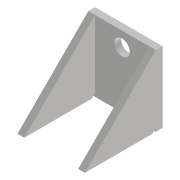
# Autodesk Inventor part: Break_tensor_support
Saved by Autodesk Inventor 2020 (Build 240168000, 168)
## iProperties
Created: 2020-02-19
Part Number: Break_tensor_support
Material: Generic
Document SubType Name: Sheet Metal
Designer: Charlie
Density: 1 g/cm^3
Sheet Metal Rule: Default_mm
Appearance: Default
Mass: 45.5555 g
Surface Area: 194.795 cm^2
Volume: 45.5555 cm^3
Author: Charlie
Autodesk Inventor part; units mm, degrees
ref_plane "YZ Plane" through (0, 0, 0) normal (1, 0, 0) x (0, 1, 0)
ref_plane "XZ Plane" through (0, 0, 0) normal (0, 1, 0) x (-1, 0, 0)
ref_plane "XY Plane" through (0, 0, 0) normal (0, 0, 1) x (1, 0, 0)
sketch "Sketch1" plane through (0, 0, 0) normal (0, 0, 1) x (1, 0, 0)
  circle A0 centre (0, 0) radius 6.85
  line L0 (-30, 13) -> (30, 13)
  line L1 (30, 13) -> (30, -50)
  line L2 (30, -50) -> (-30, -50)
  line L3 (-30, -50) -> (-30, 13)
  point P0 (0, 13)
  dimension "d0" = 13.7
  dimension "d1" = 50
  dimension "d2" = 60
  dimension "d4" = 13
  measures "d0" diameter of A0
  measures "d1" distance from line of L2 point (0, 0)
  measures "d2" distance of L0.start L0.end
  measures "d4" distance from line of L0 point (0, 0)
extrude "Plate1" add sketch "Sketch1" along normal blind 6
sketch "Sketch2" plane through (30, -50, 0) normal (1, 0, 0) x (0, 0, -1)
  line L0 (-6, 63) -> (-6, 0)
  line L1 (0, 0) -> (-6, 0)
  line L2 (0, 63) -> (0, 0)
  line L3 (0, 63) -> (-6, 63)
  line L4 (-6, 63) -> (-69, 0)
  line L5 (-69, 0) -> (-9, 0)
  line L6 (-6, 0) -> (-6, 63)
  line L7 (-6, 63) -> (-6, 3)
  line L8 (-6, 3) -> (-9, 0)
  point P0 (0, 50)
  dimension "d5" = 45
  dimension "d7" = 3
  dimension "d8" = 3
  measures "d5" angle of L5 L4
  measures "d7" distance of L7.end L0.end
  measures "d8" distance of L5.end L0.end
extrude "Plate2" add sketch "Sketch2" against normal blind 6 separate body contours L0 L8 L5 L4
mirror "Mirror1" about plane through (0, 0, 0) normal (1, 0, 0) bodies 2
equation "\"d8\" = d7"
equation "\"d3\" = Thickness"
equation "\"d6\" = Thickness"
equation "\"BendRadius\" = Thickness"
equation "\"BendReliefWidth\" = Thickness"
equation "\"BendReliefDepth\" = 0.5 * Thickness"
equation "\"CornerReliefSize\" = 4 * Thickness"
equation "\"MinimumRemnant\" = 2 * Thickness"
equation "\"TransitionRadius\" = BendRadius"
equation "\"JacobiRadiusSize\" = BendRadius"
equation "\"GapSize\" = Thickness"
equation "\"Thickness\" = 6"
